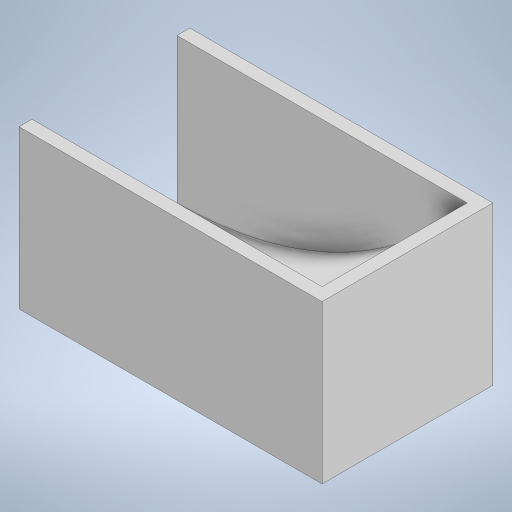
# Autodesk Inventor part: Peça que libera
Saved by Autodesk Inventor 2024 (Build 280153000, 153)
## iProperties
Created: 2023-05-16
Part Number: Peça que libera
Material: Genérico
Document SubType Name: Modeling
Designer: jpjoa
Density: 1 g/cm^3
Appearance: Padrão
Author: jpjoa
Autodesk Inventor part; units mm, degrees
ref_plane "YZ Plane" through (0, 0, 0) normal (1, 0, 0) x (0, 1, 0)
ref_plane "XZ Plane" through (0, 0, 0) normal (0, 1, 0) x (-1, 0, 0)
ref_plane "XY Plane" through (0, 0, 0) normal (0, 0, 1) x (1, 0, 0)
sketch "Esboço1" plane through (0, 0, 0) normal (0, 1, 0) x (-1, 0, 0)
  line L0 (-36, -1.6) -> (0, -1.6)
  line L1 (0, -19.6) -> (-36, -19.6)
  line L2 (-36, -19.6) -> (-36, -1.6)
  line L3 (0, 0) -> (-37.6, 0)
  line L4 (-37.6, 0) -> (-37.6, -21.2)
  line L5 (-37.6, -21.2) -> (0, -21.2)
  line L6 (0, -21.2) -> (0, 0)
  dimension "d0" = 1.6
  dimension "d1" = 18
  dimension "d7" = 36
  constraints: 14 end point, 4 perpendicular, 2 coincident, 2 point on line, 1 horizontal, 2 other
  measures "d0" distance between parallel lines of L0 L3
  measures "d1" distance of L1.end L0.start
  measures "d7" distance between parallel lines of L6 L2
sketch "Esboço1 outline for Extrusão1" plane through (0, 0, 0) normal (0, 1, 0) x (-1, 0, 0)
  line L0 (0, -21.2) -> (0, 0)
  line L1 (-37.6, -21.2) -> (0, -21.2)
  line L2 (-37.6, 0) -> (-37.6, -21.2)
  line L3 (0, 0) -> (-37.6, 0)
extrude "Extrusão1" add sketch "Esboço1 outline for Extrusão1" against normal blind 1.6
sketch "Esboço1 outline for Extrusão2" plane through (0, 0, 0) normal (0, 1, 0) x (-1, 0, 0)
  line L0 (-36, -19.6) -> (-36, -1.6)
  line L1 (0, -19.6) -> (-36, -19.6)
  line L2 (0, -21.2) -> (0, -19.6)
  line L3 (-37.6, -21.2) -> (0, -21.2)
  line L4 (-37.6, 0) -> (-37.6, -21.2)
  line L5 (0, 0) -> (-37.6, 0)
  line L6 (0, -1.6) -> (0, 0)
  line L7 (-36, -1.6) -> (0, -1.6)
extrude "Extrusão2" add sketch "Esboço1 outline for Extrusão2" along normal blind 18
fillet "Arredondamento1" radius 45 1 edges at (36, 0, -10.6)
equation "\"d0\" = Margem"
equation "\"d1\" = Esfera"
equation "\"d7\" = 2 * Esfera"
equation "\"d2\" = Margem"
equation "\"d4\" = Esfera"
equation "\"d6\" = 2.5 * Esfera"
equation "\"Esfera\" = 18"
equation "\"Margem\" = 1.6"
